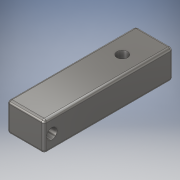
# Autodesk Inventor part: LucasCharles Part 2 arm Final
Saved by Autodesk Inventor 2018 (Build 220112000, 112)
## iProperties
Created: 2018-05-14
Part Number: LucasCharles Part 2 arm Final
Material: Stainless Steel, Austenitic
Document SubType Name: Modeling
Designer: 21lsilva
Density: 8 g/cm^3
Appearance: Semi-Polished
Author: 21lsilva
Autodesk Inventor part; units mm, degrees
ref_plane "YZ Plane" through (0, 0, 0) normal (1, 0, 0) x (0, 1, 0)
ref_plane "XZ Plane" through (0, 0, 0) normal (0, 1, 0) x (-1, 0, 0)
ref_plane "XY Plane" through (0, 0, 0) normal (0, 0, 1) x (1, 0, 0)
sketch "Sketch1" plane through (0, 0, 0) normal (0, 0, 1) x (1, 0, 0)
  line L0 (0, 0) -> (44.1452, 0)
  line L1 (44.1452, 0) -> (44.1452, 34.29)
  line L2 (44.1452, 34.29) -> (0, 34.29)
  line L3 (0, 34.29) -> (0, 0)
  dimension "d0" = 44.1452
  dimension "d1" = 34.29
  constraints: 8 end point, 2 parallel, 1 horizontal, 1 perpendicular
  measures "d0" distance of L2.end L1.end
  measures "d1" distance between parallel lines of L0 L2
extrude "Extrusion1" add sketch "Sketch1" against normal blind 152.4
sketch "Sketch3" plane through (0, 34.29, 0) normal (0, 1, 0) x (1, 0, 0)
  circle A0 centre (22.0726, 114.3) radius 6.35
  point P0 (0, 0)
  dimension "d7" = 12.7
  constraints: 1 centre point, 1 coincident
  measures "d7" diameter of A0
extrude "Extrusion3" cut sketch "Sketch3" against normal blind 50.8
sketch "Sketch4" plane through (0, 0, 0) normal (-1, 0, 0) x (0, 0, 1)
  circle A0 centre (-8.89, 17.145) radius 6.35
  line L0 (0, 34.29) -> (0, 0) projected
  point P0 (-9.5604, 26.0948)
  dimension "d14" = 12.7
  dimension "d15" = 8.89
  constraints: 1 centre point, 1 coincident
  measures "d14" diameter of A0
  measures "d15" distance from line of L0 A0.centre
extrude "Extrusion4" cut sketch "Sketch4" against normal blind 127
fillet "Fillet1" radius 3.175 11 edges at (22.0726, 0, 0) (22.0726, 34.29, 0) (44.1452, 17.145, 0) (44.1452, 34.29, -76.2) (44.1452, 0, -76.2) (44.1452, 17.145, -152.4) (0, 34.29, -76.2) (22.0726, 34.29, -152.4) (0, 17.145, -152.4) (0, 0, -76.2) (0, 17.145, 0)
fillet "Fillet2" radius 3.175 3 edges at (0.9299, 0.9299, -151.4701) (43.2153, 0.9299, -151.4701) (22.0726, 0, -152.4)
body "Solid1"
